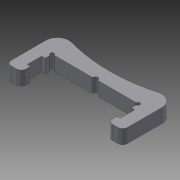
# Autodesk Inventor part: Twist Lock
Saved by Autodesk Inventor 2015 (Build 190159000, 159)
## iProperties
Created: 2015-06-17
Part Number: Twist Lock
Material: Generic
Document SubType Name: Modeling
Designer: JR
Density: 1 g/cm^3
Appearance: Default
Author: JR
Autodesk Inventor part; units mm, degrees
ref_plane "YZ Plane" through (0, 0, 0) normal (1, 0, 0) x (0, 1, 0)
ref_plane "XZ Plane" through (0, 0, 0) normal (0, 1, 0) x (-1, 0, 0)
ref_plane "XY Plane" through (0, 0, 0) normal (0, 0, 1) x (1, 0, 0)
sketch "Sketch1" plane through (0, 0, 0) normal (0, 0, 1) x (1, 0, 0)
  line L0 (0, 0) -> (-17.7, 0)
  line L1 (-20, -9.2) -> (-18.6, -9.2)
  line L2 (-18.6, -9.2) -> (-18.6, -13.2)
  line L3 (-18.6, -13.2) -> (-25, -13.2)
  line L4 (-25, -13.2) -> (-25, 3.7158)
  arc A0 (-18.6667, 8.5348) -> (-25, 3.7158) centre (-20, 3.7158) ccw
  arc A1 (-18.6667, 8.5348) -> (0, 6) centre (0, 76) ccw
  line L5 (0, 0) -> (0, 6) construction
  line L6 (-18.5, -0.8) -> (-18.5, -3)
  line L7 (-18.5, -3) -> (-20, -3)
  line L8 (-20, -3) -> (-20, -9.2)
  arc A2 (-17.7, 0) -> (-18.5, -0.8) centre (-18.5, 0) ccw
  line L9 (0, 0) -> (17.7, 0)
  line L10 (20, -9.2) -> (18.6, -9.2)
  line L11 (18.6, -9.2) -> (18.6, -13.2)
  line L12 (18.6, -13.2) -> (25, -13.2)
  line L13 (25, -13.2) -> (25, 3.7158)
  arc A3 (25, 3.7158) -> (18.6667, 8.5348) centre (20, 3.7158) ccw
  arc A4 (0, 6) -> (18.6667, 8.5348) centre (0, 76) ccw
  line L14 (18.5, -0.8) -> (18.5, -3)
  line L15 (18.5, -3) -> (20, -3)
  line L16 (20, -3) -> (20, -9.2)
  arc A5 (18.5, -0.8) -> (17.7, 0) centre (18.5, 0) ccw
  line L17 (-20, 8.7158) -> (20, 8.7158) construction
  dimension "d0" = 6
  dimension "d4" = 6.2
  dimension "d5" = 1.5
  dimension "d7" = 4
  dimension "d9" = 5
  dimension "d10" = 70
  dimension "d11" = 5
  dimension "d12" = 0.8
  dimension "d13" = 3
  dimension "d18" = 1.4
  dimension "d20" = 18.5
  dimension "d26" = 8.7158
  constraints: 36 end point, 14 point on circle, 12 symmetric about line, 6 centre point, 4 perpendicular, 4 tangent, 3 vertical, 2 horizontal, 2 vertical alignment, 1 horizontal alignment, 3 other
  measures "d0" distance of L0.start L5.end
  measures "d4" distance of L7.end L1.start
  measures "d5" distance of L6.end L7.end
  measures "d7" distance of L1.end L2.end
  measures "d9" radius of A0
  measures "d10" radius of A1
  measures "d11" distance between parallel lines of L8 L4
  measures "d12" radius of A2
  measures "d13" distance between parallel lines of L7 L0
  measures "d18" distance of L1.start L1.end
  measures "d20" distance of L0.start A2.centre
  measures "d26" distance between parallel lines of L9 L17
extrude "Extrusion1" add sketch "Sketch1" along normal blind 6
fillet "Fillet1" radius 2 4 edges at (-18.6, -13.2, 3) (-25, -13.2, 3) (18.6, -13.2, 3) (25, -13.2, 3)
fillet "Fillet2" radius 0.5 2 edges at (-18.6, -9.2, 3) (18.6, -9.2, 3)
fillet "Fillet3" radius 0.5 4 edges at (-18.5, -0.8, 3) (-17.7, 0, 3) (17.7, 0, 3) (18.5, -0.8, 3)
sketch "Sketch2" plane through (0, 0, 6) normal (0, 0, 1) x (1, 0, 0)
  arc A0 (1, 0.25) -> (-1, 0.25) centre (0, 0.25) ccw
  line L0 (-17.3, 0) -> (17.3, 0) projected
  line L1 (-1, 0.25) -> (-1, 0)
  line L2 (1, 0.25) -> (1, 0)
  point P0 (0, 0)
  point P1 (0, 0)
  dimension "d21" = 0.25
  dimension "d25" = 1
  constraints: 4 end point, 2 perpendicular, 2 point on circle, 2 point on line, 2 tangent, 1 centre point, 1 midpoint, 1 vertical alignment
  measures "d21" distance of A0.centre point (0, 0)
  measures "d25" radius of A0
extrude "Extrusion2" cut sketch "Sketch2" against normal through all
fillet "Fillet4" radius 0.5 2 edges at (-1, 0, 3) (1, 0, 3)
equation "\"d5\" = GripLength"
equation "\"d20\" = 0.5 * BattECOD - GripLength"
equation "\"GripLength\" = 1.5"
equation "\"BattECOD\" = 40"
body "Solid1"
